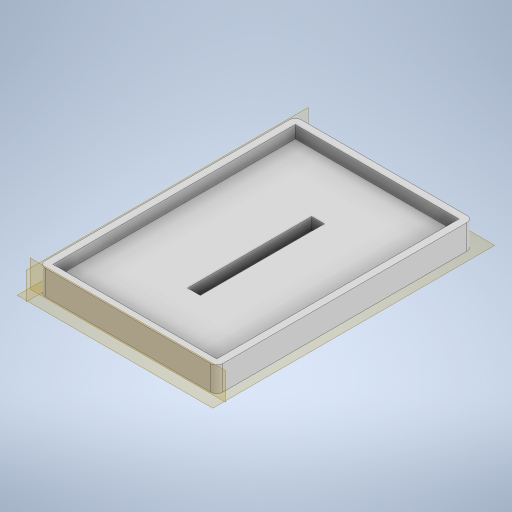
# Autodesk Inventor part: ieee_lid
Saved by Autodesk Inventor 2024 (Build 280153000, 153)
## iProperties
Created: 2023-11-14
Part Number: ieee_lid
Material: Generic
Document SubType Name: Modeling
Designer: sophi
Density: 1 g/cm^3
Appearance: Default
Author: sophi
Autodesk Inventor part; units mm, degrees
sketch "Sketch1" plane through (0, 0, 0) normal (0, 1, 0) x (-1, 0, 0)
  line L0 (0, 0) -> (-43, 0)
  line L1 (-43, 0) -> (-43, -62)
  line L2 (-43, -62) -> (0, -62)
  line L3 (0, -62) -> (0, 0)
  dimension "d0" = 43
  dimension "d1" = 62
  constraints: 8 end point, 2 parallel, 1 horizontal, 1 perpendicular
  measures "d0" distance of L1.end L2.end
  measures "d1" distance of L0.end L1.end
extrude "Extrusion1" add sketch "Sketch1" along normal blind 3
sketch "Sketch2" plane through (0, 3, 0) normal (0, 1, 0) x (1, 0, 0)
  line L0 (43, 0) -> (43, 62) projected
  line L1 (0, 0) -> (43, 0)
  line L2 (43, 0) -> (43, 62)
  line L3 (43, 62) -> (0, 62)
  line L4 (0, 62) -> (0, 0)
  line L5 (1.7, 60.3) -> (41.3, 60.3)
  line L6 (41.3, 60.3) -> (41.3, 1.7)
  line L7 (41.3, 1.7) -> (1.7, 1.7)
  line L8 (1.7, 1.7) -> (1.7, 60.3)
  dimension "d4" = 1.7
  constraints: 16 end point, 4 parallel, 2 perpendicular, 1 horizontal, 3 other
  measures "d4" distance between parallel lines of L3 L5
extrude "Extrusion2" add sketch "Sketch2" along normal blind 3
sketch "Sketch3" plane through (0, 3, 0) normal (0, 1, 0) x (1, 0, 0)
  line L0 (23.05, 46) -> (19.95, 46)
  line L1 (19.95, 46) -> (19.95, 16)
  line L2 (19.95, 16) -> (23.05, 16)
  line L3 (23.05, 16) -> (23.05, 46)
  line L4 (41.3, 60.3) -> (41.3, 1.7) projected
  line L5 (41.3, 1.7) -> (1.7, 1.7) projected
  point P0 (0, 0)
  point P1 (41.3, 31)
  point P2 (23.05, 31)
  point P3 (21.5, 1.7)
  point P4 (21.5, 16)
  dimension "d7" = 3.1
  dimension "d8" = 0
  dimension "d9" = 30
  dimension "d15" = 0
  constraints: 8 end point, 4 midpoint, 2 parallel, 1 horizontal, 1 perpendicular
  measures "d7" distance between parallel lines of L3 L1
  measures "d8" vertical distance of point (41.3, 31) point (23.05, 31)
  measures "d9" distance of L2.end L0.start
  measures "d15" horizontal distance of point (21.5, 1.7) point (21.5, 16)
extrude "Extrusion3" cut sketch "Sketch3" against normal blind 3
fillet "Fillet1" radius 1.5 4 edges at (43, 3, 0) (0, 3, 0) (0, 3, -62) (43, 3, -62)
equation "\"d0\" = width_inner + 2 * thickness"
equation "\"d1\" = length_inner + 2 * thickness"
equation "\"d2\" = thickness"
equation "\"d5\" = thickness"
equation "\"d7\" = acrylic_thickness"
equation "\"d9\" = acrylic_length"
equation "\"d11\" = thickness"
equation "\"d13\" = 0.5 * thickness"
equation "\"width_inner\" = 37"
equation "\"length_inner\" = 56"
equation "\"thickness\" = 3"
equation "\"acrylic_thickness\" = 3.1"
equation "\"acrylic_length\" = 30"
body "Solid1"
